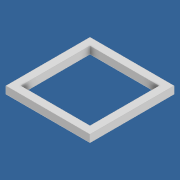
# Autodesk Inventor part: test plate
Saved by Autodesk Inventor 2020 (Build 240168000, 168)
## iProperties
Created: 2021-09-16
Part Number: test plate
Material: Generic
Document SubType Name: Modeling
Designer: RNG3nius
Density: 1 g/cm^3
Appearance: Default
Author: RNG3nius
Autodesk Inventor part; units mm, degrees
ref_plane "YZ Plane" through (0, 0, 0) normal (1, 0, 0) x (0, 1, 0)
ref_plane "XZ Plane" through (0, 0, 0) normal (0, 1, 0) x (-1, 0, 0)
ref_plane "XY Plane" through (0, 0, 0) normal (0, 0, 1) x (1, 0, 0)
sketch "Sketch1" plane through (0, 0, 0) normal (0, 1, 0) x (-1, 0, 0)
  line L0 (0, 0) -> (17, 0)
  line L1 (17, 0) -> (17, 17)
  line L2 (17, 17) -> (0, 17)
  line L3 (0, 17) -> (0, 0)
  line L4 (1.5, 1.5) -> (15.5, 1.5)
  line L5 (15.5, 1.5) -> (15.5, 15.5)
  line L6 (15.5, 15.5) -> (1.5, 15.5)
  line L7 (1.5, 15.5) -> (1.5, 1.5)
  dimension "d0" = 17
  dimension "d1" = 17
  dimension "d2" = 14
  dimension "d3" = 14
  constraints: 16 end point, 4 parallel, 2 horizontal, 2 perpendicular
  measures "d0" distance of L2.end L1.end
  measures "d1" distance of L1.end L0.end
  measures "d2" distance of L6.end L5.end
  measures "d3" distance of L5.end L4.end
extrude "Extrusion1" add sketch "Sketch1" along normal blind 1.5
body "Solid1"
